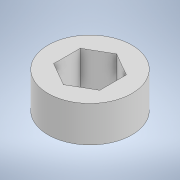
# Autodesk Inventor part: hexSpacer 3_8 x 0_300
Saved by Autodesk Inventor 2022.2 (Build 262287010, 287A)
## iProperties
Created: 2022-09-15
Part Number: hexSpacer 3_8 x 0_300
Material: Generic
Document SubType Name: Modeling
Designer: robst
Density: 1 g/cm^3
Appearance: Default
Author: robst
Autodesk Inventor part; units mm, degrees
ref_plane "YZ Plane" through (0, 0, 0) normal (1, 0, 0) x (0, 1, 0)
ref_plane "XZ Plane" through (0, 0, 0) normal (0, 1, 0) x (-1, 0, 0)
ref_plane "XY Plane" through (0, 0, 0) normal (0, 0, 1) x (1, 0, 0)
sketch "Sketch1" plane through (0, 0, 0) normal (0, 1, 0) x (-1, 0, 0)
  line L0 (4.8895, -2.823) -> (0, -5.6459)
  line L1 (0, -5.6459) -> (-4.8895, -2.823)
  line L2 (-4.8895, -2.823) -> (-4.8895, 2.823)
  line L3 (-4.8895, 2.823) -> (0, 5.6459)
  line L4 (0, 5.6459) -> (4.8895, 2.823)
  line L5 (4.8895, 2.823) -> (4.8895, -2.823)
  circle A0 centre (0, 0) radius 8.89
  dimension "d0" = 9.779
  dimension "d1" = 17.78
  constraints: 12 end point, 2 coincident, 1 centre point, 1 vertical, 13 other
  measures "d0" distance between parallel lines of L2 L5
  measures "d1" diameter of A0
extrude "Extrusion1" add sketch "Sketch1" along normal blind 7.62
body "Solid1"
